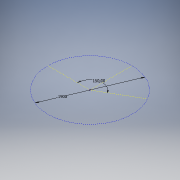
# Autodesk Inventor part: PodstawaFem
Saved by Autodesk Inventor 2017 (Build 210142000, 142)
## iProperties
Created: 2016-12-08
Part Number: PodstawaFem
Material: Generic
Document SubType Name: Modeling
Designer: Marcin
Density: 1 g/cm^3
Appearance: Default
Author: Marcin
Autodesk Inventor part; units mm, degrees
ref_plane "YZ Plane" through (0, 0, 0) normal (1, 0, 0) x (0, 1, 0)
ref_plane "XZ Plane" through (0, 0, 0) normal (0, 1, 0) x (-1, 0, 0)
ref_plane "XY Plane" through (0, 0, 0) normal (0, 0, 1) x (1, 0, 0)
sketch "Sketch1" plane through (0, 0, 0) normal (0, 1, 0) x (-1, 0, 0)
  circle A0 centre (0, 0) radius 950 construction
  line L0 (0, 0) -> (0, -950) construction
  line L1 (0, 0) -> (-822.7241, -475) construction
  line L2 (0, 0) -> (950, 0) construction
  circle A1 centre (-150, -1014.0541) radius 12.0265
  line L3 (0, 0) -> (-150, -938.0832) construction
  line L4 (-150, -938.0832) -> (-150, -1017.5235)
  dimension "d0" = 1900
  dimension "d5" = 150
  constraints: 10 end point, 2 centre point, 2 point on circle, 2 vertical, 1 coincident, 1 equal length, 1 horizontal, 1 point on line
  measures "d0" diameter of A0
  measures "d5" angle of L1 L2
extrude "Extrusion2" add sketch "Sketch1" along normal blind 80
sketch "Sketch2" plane through (150, 80, -1014.0541) normal (0, 1, 0) x (1, 0, 0)
  point P0 (-150, -1014.0541)
sketch "Sketch3" plane through (150, 80, -1014.0541) normal (0, 1, 0) x (1, 0, 0)
  line L0 (0, 0) -> (5.4512, -52.6126)
  line L1 (0, 0) -> (50.5345, 5.2359)
  point P0 (-150, -1014.0541)
  constraints: 4 end point
body "Solid2"
